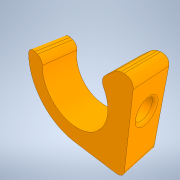
# Autodesk Inventor part: Кольцо линейного подшипника
Saved by Autodesk Inventor 2021.1 (Build 251245010, 245A)
## iProperties
Created: 2026-04-17
Part Number: Кольцо линейного подшипника
Material: Типовые
Document SubType Name: Modeling
Designer: Андрей Тарасов
Density: 1 g/cm^3
Appearance: По умолчанию
Author: Андрей Тарасов
Autodesk Inventor part; units mm, degrees
ref_plane "YZ Plane" through (0, 0, 0) normal (1, 0, 0) x (0, 1, 0)
ref_plane "XZ Plane" through (0, 0, 0) normal (0, 1, 0) x (-1, 0, 0)
ref_plane "XY Plane" through (0, 0, 0) normal (0, 0, 1) x (1, 0, 0)
sketch "Эскиз1" plane through (0, 0, 0) normal (0, 0, 1) x (1, 0, 0)
  circle A0 centre (0, 0) radius 7.6
  circle A1 centre (0, 0) radius 11.5
  line L0 (8.8095, 7.3921) -> (0, 0)
  line L1 (-16.1, 0) -> (16.1, 0) construction
  line L2 (0, 0) -> (-10.8065, 3.9332)
  line L3 (8.8095, 7.3921) -> (11.5, 7.3921)
  line L4 (11.5, 7.3921) -> (11.5, -11.5)
  line L5 (11.5, -11.5) -> (0, -11.5)
  point P0 (5.8219, 4.8852)
  point P1 (-5.8219, -4.8852)
  point P2 (-7.1417, 2.5994)
  point P3 (11.5, 0)
  dimension "d0" = 15.2
  dimension "d2" = 23
  dimension "d8" = 40
  dimension "d11" = 20
  constraints: 10 end point, 3 point on circle, 2 centre point, 2 coincident, 2 horizontal, 2 tangent, 1 midpoint, 1 perpendicular
  measures "d0" diameter of A0
  measures "d2" diameter of A1
  measures "d8" angle of L0 L1
  measures "d11" angle of L1 L2
extrude "Выдавливание1" add sketch "Эскиз1" along normal blind 8 contours A0 L0 A1 L2 | L3 L4 A1 | L4 L5 A1 picked at (-9.7933, 2.5948)
sketch "Эскиз2" plane through (0, 0, 0) normal (1, 0, 0) x (0, 1, 0)
  circle A0 centre (0, 4) radius 2.1
  line L0 (3.9332, 8) -> (-11.5, 8) projected
  line L1 (3.9332, 0) -> (-11.5, 0) projected
  line L2 (0, 8) -> (0, 0) construction
  dimension "d5" = 4.2
  constraints: 2 end point, 1 centre point, 1 midpoint, 1 perpendicular, 1 point on line
  measures "d5" diameter of A0
extrude "Выдавливание2" cut sketch "Эскиз2" along normal blind 15
fillet "Сопряжение1" radius 1.6 6 edges at (8.8095, 7.3921, 4) (5.8219, 4.8852, 4) (-7.1417, 2.5994, 4) (-10.8065, 3.9332, 4) (11.5, 7.3921, 4) (11.5, -11.5, 4)
fillet "Сопряжение1" radius 0.6 2 edges at (7.3041, -2.1, 4.0117) (11.5, -2.1, 4)
